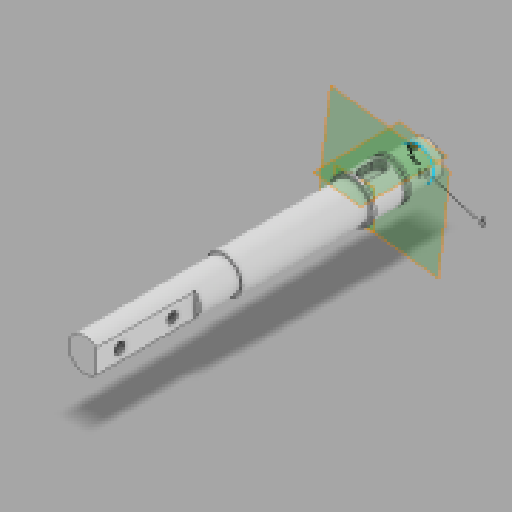
# Autodesk Inventor part: Вал вертикальной оси
Saved by Autodesk Inventor 2025 (Build 290162000, 162)
## iProperties
Created: 2025-04-08
Part Number: Вал вертикальной оси
Material: Типовые
Document SubType Name: Modeling
Designer: Artem Sannikov
Density: 1 g/cm^3
Appearance: По умолчанию
Author: Artem Sannikov
Autodesk Inventor part; units mm, degrees
ref_plane "YZ Plane" through (0, 0, 0) normal (1, 0, 0) x (0, 1, 0)
sketch "Эскиз1" plane through (0, 0, 0) normal (0, 0, 1) x (1, 0, 0)
  arc A0 (0.3914, -1.6228) -> (0.394, 1.6268) centre (2.903, 0) ccw construction
  circle A1 centre (2.903, 0) radius 2.9903
  circle A2 centre (2.903, 0) radius 6
  point P0 (0, 0)
  dimension "d0" = 12
  constraints: 2 centre point, 2 coincident, 1 concentric
  measures "d0" diameter of A2
extrude "Выдавливание1" add sketch "Эскиз1" along normal blind 24
ref_plane "РабПлоскость2" through (3.6207, 5.9569, 0) normal (-0.1196, -0.9928, 0) x (0.9928, -0.1196, 0)
ref_plane "РабПлоскость1" through (5.8216, 7.5048, 10) normal (-0.1196, -0.9928, 0) x (0.9928, -0.1196, 0)
sketch "Эскиз2" plane through (3.6207, 5.9569, 0) normal (-0.1196, -0.9928, 0) x (0.9928, -0.1196, 0)
  line L0 (6, 0) -> (-6, 0) projected
  line L1 (0, 0) -> (0, 19.3984) construction
  line L2 (0, 12.5) -> (0, 16.5) construction
  line L3 (2, 12.5) -> (2, 16.5)
  line L4 (-2, 16.5) -> (-2, 12.5)
  arc A0 (-2, 12.5) -> (2, 12.5) centre (0, 12.5) ccw
  arc A1 (2, 16.5) -> (-2, 16.5) centre (0, 16.5) ccw
  point P0 (-2.8822, 0)
  point P1 (0, 14.5)
  dimension "d0" = 12
  dimension "d3" = 4
  dimension "d4" = 4
  dimension "d5" = 14.5
  constraints: 10 end point, 4 point on circle, 4 tangent, 2 centre point, 2 midpoint, 2 point on line, 1 parallel, 1 vertical
  measures "d3" distance of L2.start L2.end
  measures "d4" diameter of A1
  measures "d5" distance of L1.start point (0, 14.5)
extrude "Выдавливание2" cut sketch "Эскиз2" along normal blind 2.5
ref_plane "РабПлоскость3" through (2.903, 0, 19) normal (0, 0, -1) x (-1, 0, 0)
sketch "Эскиз3" plane through (2.903, 0, 19) normal (0, 0, -1) x (-1, 0, 0)
  point P0 (2.903, 0)
sketch "Эскиз4" plane through (2.903, 0, 19) normal (0, 0, -1) x (-1, 0, 0)
  circle A0 centre (0, 0) radius 6.5
  point P0 (2.903, 0)
  dimension "d12" = 13
  constraints: 1 centre point
  measures "d12" diameter of A0
extrude "Выдавливание3" add sketch "Эскиз4" against normal blind 20
sketch "Эскиз5" plane through (2.903, 0, 39) normal (0, 0, 1) x (1, 0, 0)
  circle A0 centre (0, 0) radius 5
  circle A1 centre (0, 0) radius 7.2744
  point P0 (-2.903, 0)
  dimension "d15" = 10
  constraints: 2 centre point, 1 coincident
  measures "d15" diameter of A0
extrude "Выдавливание4" cut sketch "Эскиз5" against normal blind 19
sketch "Эскиз6" plane through (2.903, 0, 0) normal (0, 0, -1) x (-1, 0, 0)
  circle A0 centre (0, 0) radius 3
  circle A1 centre (0, 0) radius 5
  point P0 (2.903, 0)
  dimension "d18" = 6
  dimension "d19" = 10
  constraints: 2 centre point, 1 coincident
  measures "d18" diameter of A0
  measures "d19" diameter of A1
ref_plane "РабПлоскость4" through (-4.5219, -7.4249, -3) normal (0, 0, 1) x (1, 0, 0)
sketch "Эскиз8" plane through (2.903, 0, 0) normal (0, 0, -1) x (-1, 0, 0)
  circle A0 centre (0, 0) radius 6 projected
  point P0 (2.903, 0)
extrude "Выдавливание6" cut sketch "Эскиз8" against normal blind 9
sketch "Эскиз9" plane through (2.903, 0, 9) normal (0, 0, -1) x (-1, 0, 0)
  circle A0 centre (0, 0) radius 3
  circle A1 centre (0, 0) radius 5
  point P0 (2.903, 0)
  dimension "d24" = 6
  dimension "d25" = 10
  constraints: 2 centre point, 1 coincident
  measures "d24" diameter of A0
  measures "d25" diameter of A1
ref_plane "РабПлоскость5" through (-4.5219, -7.4249, -3) normal (0, 0, 1) x (1, 0, 0)
extrude "Выдавливание7" add sketch "Эскиз9" along normal up to surface (12 mm away)
sketch "Эскиз10" plane through (2.903, 0, 39) normal (0, 0, 1) x (1, 0, 0)
  circle A0 centre (0, 0) radius 5
  point P0 (-2.903, 0)
  constraints: 1 centre point
extrude "Выдавливание8" add sketch "Эскиз10" along normal blind 62
sketch "Эскиз11" plane through (2.903, 0, 101) normal (0, 0, 1) x (1, 0, 0)
  line L0 (3.5, 4.5942) -> (9.6944, 4.5942)
  line L1 (9.6944, 4.5942) -> (9.6944, -5.4033)
  line L2 (9.6944, -5.4033) -> (3.5, -5.4033)
  line L3 (3.5, -5.4033) -> (3.5, 4.5942)
  circle A0 centre (0, 0) radius 5 projected
  point P0 (-2.903, 0)
  point P1 (3.5, 3.5707)
  point P2 (3.5, -3.5707)
  dimension "d30" = 3.5
  constraints: 8 end point, 2 parallel, 1 horizontal, 1 perpendicular
  measures "d30" distance from line of A0.centre L3
extrude "Выдавливание9" cut sketch "Эскиз11" against normal blind 30 contours A0 L3 picked at (3.7121, 0.9363)
sketch "Эскиз12" plane through (2.903, 0, 20) normal (0, 0, 1) x (1, 0, 0)
  circle A0 centre (0, 0) radius 5.5
  point P0 (-2.903, 0)
  dimension "d33" = 11
  constraints: 1 centre point
  measures "d33" diameter of A0
extrude "Выдавливание10" add sketch "Эскиз12" along normal blind 38.8
sketch "Эскиз13" plane through (6.403, -3.5707, 101) normal (1, 0, 0) x (0, 0, -1)
  point P0 (101, 3.5707)
sketch "Эскиз14" plane through (6.403, -3.5707, 101) normal (1, 0, 0) x (0, 0, -1)
  point P0 (101, 3.5707)
sketch "Эскиз15" plane through (6.403, -3.5707, 101) normal (1, 0, 0) x (0, 0, -1)
  line L0 (30, 0) -> (30, 7.1414) projected
  line L1 (30, 3.5707) -> (0, 3.5707) construction
  line L2 (0, 8.5707) -> (0, -1.4293) projected
  point P0 (101, 3.5707)
  point P1 (0, 7.1414)
  point P2 (0, 0)
  point P3 (7, 3.5707)
  point P4 (23, 3.5707)
  dimension "d36" = 7
  dimension "d37" = 7
  constraints: 2 end point, 2 midpoint, 2 point on line
  measures "d36" distance from line of L2 point (7, 3.571)
  measures "d37" distance from line of L0 point (23, 3.571)
hole "Отверстие1" at (6.403, 0, 94) at (6.403, 0, 78) direction (-1, 0, 0) diameter 3.242 depth 11.8 tip angle 118 thread size "M4x0.7" class "6H" standard "ISO Metric profile"
sketch "Эскиз16" plane through (2.903, 0, 9) normal (0, 0, -1) x (-1, 0, 0)
  circle A0 centre (0, 0) radius 6 projected
  point P0 (2.903, 0)
extrude "Выдавливание11" add sketch "Эскиз16" along normal blind 1
ref_plane "РабПлоскость6" through (2.903, 0, 10) normal (0, 0, -1) x (0.9928, -0.1196, 0)
sketch "Эскиз17" plane through (2.903, 0, 10) normal (0, 0, -1) x (0.9928, -0.1196, 0)
  circle A0 centre (0, 0) radius 5.65
  circle A1 centre (0, 0) radius 7.5447
  point P0 (-2.8822, 0.3472)
  dimension "d47" = 11.3
  constraints: 2 centre point, 1 coincident
  measures "d47" diameter of A0
extrude "Выдавливание12" cut sketch "Эскиз17" along normal blind 1.2
sketch "Эскиз18" plane through (0, 0, 0) normal (0, 1, 0) x (-1, 0, 0)
  line L0 (-7.903, -3) -> (2.097, -3) construction
  line L1 (2.097, -3) -> (-7.903, -3)
  line L2 (-2.903, -3) -> (-2.903, 1.2) construction
  point P0 (0, 0)
  dimension "d50" = 4.2
  constraints: 4 end point, 2 coincident, 1 horizontal, 1 midpoint, 1 vertical
  measures "d50" distance of L2.start L2.end
hole "Отверстие2" at (2.903, 0, 1.2) direction (0, 1, 0) diameter 2.459 depth 8.8 tip angle 118 thread size "M3x0.5" class "6H" standard "ISO Metric profile"
